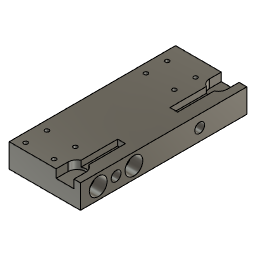
seitenteil links v17 (Autodesk Fusion 360 design; units mm, degrees)
Autodesk Fusion 360 part; units mm, degrees
sketch "Skizze1" plane through (0, 0, 0) normal (0, 0, 1) x (1, 0, 0)
  line L0 (0, 0) -> (60, 0)
  line L1 (60, 0) -> (60, 140)
  line L2 (60, 140) -> (0, 140)
  line L3 (0, 140) -> (0, 0)
  dimension "d1" = 60
  dimension "d2" = 140
  constraint horizontal L0
  constraint vertical L1
  constraint horizontal L2
  constraint vertical L3
  constraint coincident L0.start L3.end
  measures "d1" distance of L0.start L0.end
  measures "d2" distance of L0.start L2.end
extrude "Extrusion1" add sketch "Skizze1" along normal blind 20
sketch "Skizze2" plane through (60, 0, 0) normal (1, 0, 0) x (0, 1, 0)
  line L0 (0, 0) -> (140, 0)
  line L1 (140, 0) -> (140, 20)
  line L2 (140, 20) -> (0, 20)
  line L3 (0, 20) -> (0, 0)
  circle A0 centre (30, 10) radius 4.15
  circle A1 centre (100.3, 10) radius 4.15
  point P0 (0, 10)
  dimension "d5" = 8.3
  dimension "d6" = 8.3
  constraint midpoint L3 P0
  constraint horizontal A0.centre P0
  constraint horizontal P0 A1.centre
  measures "d5" diameter of A0
  measures "d6" diameter of A1
extrude "Extrusion2" cut sketch "Skizze2" against normal blind 50 contours A0 | A1
sketch "Skizze3" plane through (0, 0, 20) normal (0, 0, 1) x (-1, 0, 0)
  line L0 (0, -140) -> (0, 0)
  line L1 (0, 0) -> (-60, 0)
  line L2 (-60, 0) -> (-60, -140)
  line L3 (-60, -140) -> (0, -140)
  circle A0 centre (-31.6, -24.1) radius 1.7
  circle A1 centre (-7.7, -24.1) radius 1.7
  circle A2 centre (-31.6, -6.2) radius 1.7
  circle A3 centre (-7.7, -6.2) radius 1.7
  circle A4 centre (-7.7, -107.4) radius 1.7
  circle A5 centre (-31.6, -125.3) radius 1.7
  circle A6 centre (-7.7, -125.3) radius 1.7
  circle A7 centre (-31.6, -107.4) radius 1.7
  dimension "d9" = 3.4
  dimension "d10" = 3.4
  dimension "d11" = 3.4
  dimension "d12" = 3.4
  dimension "d13" = 3.4
  dimension "d14" = 3.4
  dimension "d15" = 3.4
  dimension "d16" = 3.4
  measures "d9" diameter of A0
  measures "d10" diameter of A1
  measures "d11" diameter of A2
  measures "d12" diameter of A3
  measures "d13" diameter of A4
  measures "d14" diameter of A5
  measures "d15" diameter of A6
  measures "d16" diameter of A7
extrude "Extrusion3" cut sketch "Skizze3" against normal blind 20 contours A0 | A1 | A2 | A3 | A4 | A5 | A6 | A7
sketch "Skizze5" plane through (0, 0, 0) normal (0, 0, -1) x (1, 0, 0)
  line L0 (0, 0) -> (0, -140)
  line L1 (0, -140) -> (60, -140)
  line L2 (60, -140) -> (60, 0)
  line L3 (60, 0) -> (0, 0)
  circle A0 centre (46, -130) radius 1
  circle A1 centre (7.7, -125.3) radius 1.7
  circle A2 centre (31.6, -24.1) radius 1.7
  circle A3 centre (31.6, -6.2) radius 1.7
  circle A4 centre (31.6, -125.3) radius 1.7
  circle A5 centre (7.7, -107.4) radius 1.7
  circle A6 centre (7.7, -24.1) radius 1.7
  circle A7 centre (7.7, -6.2) radius 1.7
  circle A8 centre (31.6, -107.4) radius 1.7
  dimension "d22" = 2
  measures "d22" diameter of A0
sketch "Skizze6" plane through (0, 0, 0) normal (0, 0, -1) x (1, 0, 0)
  circle A0 centre (7.7, -125.3) radius 1.7
  circle A1 centre (31.6, -24.1) radius 1.7
  circle A2 centre (31.6, -6.2) radius 1.7
  circle A3 centre (31.6, -125.3) radius 1.7
  circle A4 centre (7.7, -107.4) radius 1.7
  circle A5 centre (7.7, -24.1) radius 1.7
  circle A6 centre (7.7, -6.2) radius 1.7
  circle A7 centre (31.6, -107.4) radius 1.7
  line L0 (0, 0) -> (0, -140)
  line L1 (0, -140) -> (60, -140)
  line L2 (60, -140) -> (60, 0)
  line L3 (60, 0) -> (0, 0)
  line L4 (60, -53.1468) -> (40, -53.1468)
  line L5 (40, -53.1468) -> (40, -85.1468)
  line L6 (40, -85.1468) -> (60, -85.1468)
  line L7 (60, -85.1468) -> (60, -53.1468)
  line L8 (60, -53.1468) -> (40, -53.1468)
  line L9 (40, -53.1468) -> (40, -58.1468)
  line L10 (40, -58.1468) -> (60, -58.1468)
  line L11 (60, -58.1468) -> (60, -53.1468)
  line L12 (40, -85.1468) -> (60, -85.1468)
  line L13 (60, -85.1468) -> (60, -80.1468)
  line L14 (60, -80.1468) -> (40, -80.1468)
  line L15 (40, -80.1468) -> (40, -85.1468)
  line L16 (53.5, -63.5) -> (36.5, -63.5)
  arc A8 (36.5, -63.5) -> (36.5, -66.5) centre (36.5, -65) ccw
  line L17 (36.5, -66.5) -> (53.5, -66.5)
  arc A9 (53.5, -66.5) -> (53.5, -63.5) centre (53.5, -65) ccw
  line L18 (55, -65) -> (35, -65) construction
  line L19 (36.5, -75.4708) -> (53.5, -75.4708)
  arc A10 (53.5, -75.4708) -> (53.5, -72.4708) centre (53.5, -73.9708) ccw
  line L20 (53.5, -72.4708) -> (36.5, -72.4708)
  arc A11 (36.5, -72.4708) -> (36.5, -75.4708) centre (36.5, -73.9708) ccw
  line L21 (35, -73.9708) -> (55, -73.9708) construction
  dimension "d31" = 20
  dimension "d32" = 32
  dimension "d33" = 20
  dimension "d34" = 5
  dimension "d35" = 20
  dimension "d36" = 5
  dimension "d72" = 3
  dimension "d73" = 3
  constraint horizontal L4
  constraint vertical L5
  constraint horizontal L6
  constraint vertical L7
  constraint coincident L2 L4.start
  constraint horizontal L8
  constraint vertical L9
  constraint horizontal L10
  constraint vertical L11
  constraint horizontal L12
  constraint vertical L13
  constraint horizontal L14
  constraint vertical L15
  constraint tangent L16 A8
  constraint tangent A8 L17
  constraint parallel L16 L17
  constraint tangent L17 A9
  constraint tangent L16 A9
  constraint midpoint A9 L18.start
  constraint midpoint A8 L18.end
  constraint perpendicular L5 L18
  constraint tangent L19 A10
  constraint tangent A10 L20
  constraint parallel L19 L20
  constraint tangent L20 A11
  constraint tangent L19 A11
  constraint midpoint A11 L21.start
  constraint midpoint A10 L21.end
  constraint horizontal L21
  measures "d31" distance of L4.start L4.end
  measures "d32" distance of L4.start L6.end
  measures "d33" distance of L4.start L4.end
  measures "d34" distance of L4.start L10.end
  measures "d35" distance of L5.end L6.end
  measures "d36" distance of L5.end L14.end
  measures "d72" diameter of A8
  measures "d73" diameter of A10
extrude "Extrusion19" cut sketch "Skizze6" against normal blind 1 contours L5 L16 L17 A9 | L5 L16 A8 L17 | L5 L19 L20 A11 | L5 L19 A10 L20
extrude "Extrusion7" add sketch "Skizze6" along normal blind 12 contours L2 L4 L5 L7 L8 L9 L10 L11 | L2 L5 L6 L7 L12 L13 L14 L15
sketch "Skizze8" plane through (0, 0, 0) normal (-1, 0, 0) x (0, -1, 0)
  line L0 (-140, 0) -> (0, 0)
  line L1 (0, 0) -> (0, 20)
  line L2 (0, 20) -> (-140, 20)
  line L3 (-140, 20) -> (-140, 0)
  circle A0 centre (-15, 10) radius 2.2
  circle A1 centre (-45, 10) radius 2.2
  dimension "d27" = 4.4
  dimension "d28" = 4.4
  measures "d27" diameter of A0
  measures "d28" diameter of A1
extrude "Extrusion6" cut sketch "Skizze8" against normal blind 60 contours A0 | A1
sketch "Skizze10" plane through (60, 0, 0) normal (1, 0, 0) x (0, 1, 0)
  line L0 (58.1468, -12) -> (58.1468, 0)
  line L1 (58.1468, 0) -> (80.1468, 0)
  line L2 (80.1468, 0) -> (80.1468, -12)
  circle A0 centre (15, 10) radius 2.2
  circle A1 centre (45, 10) radius 2.2
  circle A2 centre (30, 10) radius 4.15
  circle A3 centre (100.3, 10) radius 4.15
  line L3 (53.1468, -12) -> (58.1468, -12)
  line L4 (85.1468, -12) -> (85.1468, 0)
  line L5 (85.1468, 0) -> (140, 0)
  line L6 (140, 0) -> (140, 20)
  line L7 (140, 20) -> (0, 20)
  line L8 (0, 20) -> (0, 0)
  line L9 (0, 0) -> (53.1468, 0)
  line L10 (53.1468, 0) -> (53.1468, -12)
  circle A4 centre (15, 10) radius 7.5
  circle A5 centre (45, 10) radius 7.5
  line L11 (80.1468, -12) -> (85.1468, -12)
  dimension "d42" = 15
  dimension "d43" = 15
  constraint concentric A0 A4
  constraint concentric A1 A5
  measures "d42" diameter of A4
  measures "d43" diameter of A5
extrude "Extrusion9" cut sketch "Skizze10" against normal blind 10 contours A4 | A5
sketch "Skizze13" plane through (0, 0, 20) normal (0, 0, 1) x (-1, 0, 0)
  circle A0 centre (-7.7, -125.3) radius 1.7
  circle A1 centre (-31.6, -24.1) radius 1.7
  circle A2 centre (-31.6, -6.2) radius 1.7
  circle A3 centre (-31.6, -125.3) radius 1.7
  circle A4 centre (-7.7, -107.4) radius 1.7
  circle A5 centre (-7.7, -24.1) radius 1.7
  circle A6 centre (-7.7, -6.2) radius 1.7
  circle A7 centre (-31.6, -107.4) radius 1.7
  line L0 (0, -140) -> (0, 0)
  line L1 (0, 0) -> (-60, 0)
  line L2 (-60, 0) -> (-60, -140)
  line L3 (-60, -140) -> (0, -140)
  circle A8 centre (-47, -10) radius 7.5
  dimension "d53" = 15
  measures "d53" diameter of A8
extrude "Extrusion12" cut sketch "Skizze13" against normal blind 5 contours A8
sketch "Skizze14" plane through (0, 0, 15) normal (0, 0, 1) x (-1, 0, 0)
  line L0 (-50, -9.4098) -> (-50, -16.8739)
  arc A0 (-50, -16.8739) -> (-54.4767, -9.4098) centre (-47, -10) ccw
  line L1 (-54.4767, -9.4098) -> (-50, -9.4098)
  circle A1 centre (-47, -10) radius 1
  dimension "d56" = 2
  constraint concentric A0 A1
  measures "d56" diameter of A1
extrude "Extrusion13" cut sketch "Skizze14" against normal blind 1 contours A1
sketch "Skizze15" plane through (0, 0, 20) normal (0, 0, 1) x (-1, 0, 0)
  circle A0 centre (-47, -10) radius 7.5
  circle A1 centre (-7.7, -125.3) radius 1.7
  circle A2 centre (-31.6, -24.1) radius 1.7
  circle A3 centre (-31.6, -6.2) radius 1.7
  circle A4 centre (-31.6, -125.3) radius 1.7
  circle A5 centre (-7.7, -107.4) radius 1.7
  circle A6 centre (-7.7, -24.1) radius 1.7
  circle A7 centre (-7.7, -6.2) radius 1.7
  circle A8 centre (-31.6, -107.4) radius 1.7
  line L0 (0, -140) -> (0, 0)
  line L1 (0, 0) -> (-60, 0)
  line L2 (-60, 0) -> (-60, -140)
  line L3 (-60, -140) -> (0, -140)
  line L4 (-39.5, 0) -> (-54.5, 0)
  line L5 (-54.5, 0) -> (-54.5, -17.5)
  line L6 (-54.5, -17.5) -> (-39.5, -17.5)
  line L7 (-39.5, -17.5) -> (-39.5, 0)
  constraint horizontal L4
  constraint vertical L5
  constraint horizontal L6
  constraint vertical L7
  constraint coincident L1 L4.start
  constraint tangent A0 L7
  constraint tangent A0 L5
  constraint tangent A0 L6
extrude "Extrusion14" cut sketch "Skizze15" against normal blind 7 contours A0 | A0 L1 L4 L5 L7
sketch "Skizze16" plane through (0, 0, 20) normal (0, 0, 1) x (-1, 0, 0)
  circle A0 centre (-31.6, -107.4) radius 1.7
  circle A1 centre (-7.7, -6.2) radius 1.7
  circle A2 centre (-7.7, -24.1) radius 1.7
  circle A3 centre (-7.7, -107.4) radius 1.7
  circle A4 centre (-31.6, -125.3) radius 1.7
  circle A5 centre (-31.6, -6.2) radius 1.7
  circle A6 centre (-31.6, -24.1) radius 1.7
  circle A7 centre (-7.7, -125.3) radius 1.7
  line L0 (-39.5, 0) -> (-39.5, -10)
  arc A8 (-54.5, -10) -> (-39.5, -10) centre (-47, -10) ccw
  line L1 (-54.5, -10) -> (-54.5, 0)
  line L2 (-54.5, 0) -> (-60, 0)
  line L3 (-60, 0) -> (-60, -140)
  line L4 (-60, -140) -> (0, -140)
  line L5 (0, -140) -> (0, 0)
  line L6 (0, 0) -> (-39.5, 0)
  circle A9 centre (-46, -130) radius 7.5
  line L7 (-38.5, -140) -> (-53.5, -140)
  line L8 (-53.5, -140) -> (-53.5, -122.5)
  line L9 (-53.5, -122.5) -> (-38.5, -122.5)
  line L10 (-38.5, -122.5) -> (-38.5, -140)
  dimension "d61" = 15
  constraint horizontal L7
  constraint vertical L8
  constraint horizontal L9
  constraint vertical L10
  constraint coincident L4 L7.start
  constraint tangent A9 L8
  constraint tangent A9 L9
  constraint tangent A9 L10
  measures "d61" diameter of A9
extrude "Extrusion15" cut sketch "Skizze16" against normal blind 7 contours L4 A9 L7 L8 L10 | A9
sketch "Skizze17" plane through (0, 0, 20) normal (0, 0, 1) x (-1, 0, 0)
  line L0 (-38.5, -130) -> (-38.5, -140)
  line L1 (-38.5, -140) -> (0, -140)
  line L2 (0, -140) -> (0, 0)
  line L3 (0, 0) -> (-39.5, 0)
  line L4 (-39.5, 0) -> (-39.5, -10)
  arc A0 (-54.5, -10) -> (-39.5, -10) centre (-47, -10) ccw
  line L5 (-54.5, -10) -> (-54.5, 0)
  line L6 (-54.5, 0) -> (-60, 0)
  line L7 (-60, 0) -> (-60, -140)
  line L8 (-60, -140) -> (-53.5, -140)
  line L9 (-53.5, -140) -> (-53.5, -130)
  arc A1 (-38.5, -130) -> (-53.5, -130) centre (-46, -130) ccw
  circle A2 centre (-31.6, -107.4) radius 1.7
  circle A3 centre (-7.7, -6.2) radius 1.7
  circle A4 centre (-7.7, -24.1) radius 1.7
  circle A5 centre (-7.7, -107.4) radius 1.7
  circle A6 centre (-31.6, -125.3) radius 1.7
  circle A7 centre (-31.6, -6.2) radius 1.7
  circle A8 centre (-31.6, -24.1) radius 1.7
  circle A9 centre (-7.7, -125.3) radius 1.7
  line L10 (-49.25, -92.5) -> (-42.75, -92.5)
  line L11 (-42.75, -92.5) -> (-42.75, -152.5)
  line L12 (-42.75, -152.5) -> (-49.25, -152.5)
  line L13 (-49.25, -152.5) -> (-49.25, -92.5)
  line L14 (-49.25, -92.5) -> (-42.75, -152.5) construction
  line L15 (-42.75, -92.5) -> (-49.25, -152.5) construction
  point P0 (-46, -122.5)
  dimension "d64" = 60
  dimension "d65" = 6.5
  constraint perpendicular L10 L11
  constraint parallel L10 L12
  constraint parallel L11 L13
  constraint horizontal L10
  constraint coincident L14 P0
  constraint coincident L15 P0
  constraint midpoint A1 P0
  measures "d64" distance of L10.end L11.end
  measures "d65" distance of L11.end L12.end
extrude "Extrusion16" cut sketch "Skizze17" against normal blind 5 contours A1 L10 L11 L13
sketch "Skizze18" plane through (0, 0, 20) normal (0, 0, 1) x (-1, 0, 0)
  line L0 (-42.75, -92.5) -> (-42.75, -123.2407)
  arc A0 (-38.5, -130) -> (-42.75, -123.2407) centre (-46, -130) ccw
  line L1 (-38.5, -130) -> (-38.5, -140)
  line L2 (-38.5, -140) -> (0, -140)
  line L3 (0, -140) -> (0, 0)
  line L4 (0, 0) -> (-39.5, 0)
  line L5 (-39.5, 0) -> (-39.5, -10)
  arc A1 (-54.5, -10) -> (-39.5, -10) centre (-47, -10) ccw
  line L6 (-54.5, -10) -> (-54.5, 0)
  line L7 (-54.5, 0) -> (-60, 0)
  line L8 (-60, 0) -> (-60, -140)
  line L9 (-60, -140) -> (-53.5, -140)
  line L10 (-53.5, -140) -> (-53.5, -130)
  arc A2 (-49.25, -123.2407) -> (-53.5, -130) centre (-46, -130) ccw
  line L11 (-49.25, -123.2407) -> (-49.25, -92.5)
  line L12 (-49.25, -92.5) -> (-42.75, -92.5)
  circle A3 centre (-31.6, -107.4) radius 1.7
  circle A4 centre (-7.7, -6.2) radius 1.7
  circle A5 centre (-7.7, -24.1) radius 1.7
  circle A6 centre (-7.7, -107.4) radius 1.7
  circle A7 centre (-31.6, -125.3) radius 1.7
  circle A8 centre (-31.6, -6.2) radius 1.7
  circle A9 centre (-31.6, -24.1) radius 1.7
  circle A10 centre (-7.7, -125.3) radius 1.7
  line L13 (-50.25, -47.5) -> (-43.75, -47.5)
  line L14 (-43.75, -47.5) -> (-43.75, 12.5)
  line L15 (-43.75, 12.5) -> (-50.25, 12.5)
  line L16 (-50.25, 12.5) -> (-50.25, -47.5)
  line L17 (-50.25, -47.5) -> (-43.75, 12.5) construction
  line L18 (-43.75, -47.5) -> (-50.25, 12.5) construction
  point P0 (-47, -17.5)
  dimension "d68" = 6.5
  dimension "d69" = 60
  constraint perpendicular L13 L14
  constraint parallel L13 L15
  constraint parallel L14 L16
  constraint horizontal L13
  constraint coincident L17 P0
  constraint coincident L18 P0
  constraint midpoint A1 P0
  measures "d68" distance of L14.end L15.end
  measures "d69" distance of L13.end L14.end
extrude "Extrusion17" cut sketch "Skizze18" against normal blind 5 contours A1 L13 L14 L16
extrude "Extrusion18" cut 2 faces at (46.6667, 54.8135, -12) (53.3333, 83.4802, -12) along direction (0, 0, 1) blind 12
